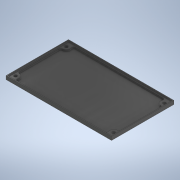
# Autodesk Inventor part: SUSTAINA-Core-Board_cover
Saved by Autodesk Inventor 2022.3 (Build 263350000, 350)
## iProperties
Part Number: SUSTAINA-Core-Board_cover
Material: 一般
Document SubType Name: Modeling
Designer: Masato Kubotera
Density: 1 g/cm^3
Appearance: 濃い灰色
Description: PLA
Mass: 6.13737 g
Surface Area: 193.634 cm^2
Volume: 6.13737 cm^3
Author: Masato Kubotera
Autodesk Inventor part; units mm, degrees
ref_plane "YZ Plane" through (0, 0, 0) normal (1, 0, 0) x (0, 1, 0)
ref_plane "XZ Plane" through (0, 0, 0) normal (0, 1, 0) x (-1, 0, 0)
derived "MainBoard.ipt"
sketch "スケッチ3" plane through (0, 0, -88.5) normal (0, 0, 1) x (1, 0, 0)
  line L0 (20.25, -135) -> (20.25, 0)
  line L1 (-83.25, 0) -> (-83.25, -135)
  line L2 (-31.5, -135) -> (-31.5, 0) construction
  line L3 (-83.25, -67.5) -> (20.25, -67.5) construction
  line L4 (-52.45, 1.4849) -> (-52.45, 5)
  line L5 (-52.45, 5) -> (-10.55, 5)
  line L6 (-10.55, 5) -> (-10.55, 1.4849)
  arc A0 (-53.9349, 0) -> (-52.45, 1.4849) centre (-53.1925, 0.7425) ccw
  arc A1 (-10.55, 1.4849) -> (-9.0651, 0) centre (-9.8075, 0.7425) ccw
  line L7 (-53.9349, 0) -> (-83.25, 0)
  line L8 (20.25, 0) -> (-9.0651, 0)
  line L9 (-10.55, 0) -> (-52.45, 0)
  line L10 (-52.45, -136.4849) -> (-52.45, -140)
  line L11 (-52.45, -140) -> (-10.55, -140)
  line L12 (-10.55, -140) -> (-10.55, -136.4849)
  arc A2 (-52.45, -136.4849) -> (-53.9349, -135) centre (-53.1925, -135.7425) ccw
  arc A3 (-9.0651, -135) -> (-10.55, -136.4849) centre (-9.8075, -135.7425) ccw
  line L13 (-53.9349, -135) -> (-83.25, -135)
  line L14 (20.25, -135) -> (-9.0651, -135)
  line L15 (-10.55, -135) -> (-52.45, -135)
  line L16 (18, -127.5) -> (-52, -127.5) construction
  line L17 (-52, -127.5) -> (-52, -7.5) construction
  line L18 (-52, -7.5) -> (18, -7.5) construction
  line L19 (18, -7.5) -> (18, -127.5) construction
  line L20 (18, -127.5) -> (-52, -7.5) construction
  line L21 (-52, -127.5) -> (18, -7.5) construction
  line L22 (-48.5, -116.5) -> (-48.5, -18.5)
  line L23 (-38.5627, -9.5) -> (4.5627, -9.5)
  line L24 (12.5, -10.5) -> (-46.5, -10.5) construction
  line L25 (-46.5, -10.5) -> (-46.5, -124.5) construction
  line L26 (-46.5, -124.5) -> (12.5, -124.5) construction
  line L27 (12.5, -124.5) -> (12.5, -10.5) construction
  line L28 (12.5, -10.5) -> (-46.5, -124.5) construction
  line L29 (-46.5, -10.5) -> (12.5, -124.5) construction
  circle A4 centre (12.5, -10.5) radius 2
  circle A5 centre (-46.5, -10.5) radius 2
  arc A6 (-46.5, -16.5) -> (-40.5471, -11.25) centre (-46.5, -10.5) ccw
  arc A7 (6.5471, -11.25) -> (12.5, -16.5) centre (12.5, -10.5) ccw
  line L30 (14.5, -18.5) -> (14.5, -116.5)
  line L31 (-17, -7.5) -> (-17, -127.5) construction
  line L32 (-76.25, -65) -> (-56.5, -65)
  line L33 (-54.5, -63) -> (-54.5, -7)
  line L34 (-56.5, -5) -> (-76.25, -5)
  line L35 (-78.25, -7) -> (-78.25, -63)
  arc A8 (-78.25, -63) -> (-76.25, -65) centre (-76.25, -63) ccw
  arc A9 (-56.5, -65) -> (-54.5, -63) centre (-56.5, -63) ccw
  arc A10 (-54.5, -7) -> (-56.5, -5) centre (-56.5, -7) ccw
  arc A11 (-76.25, -5) -> (-78.25, -7) centre (-76.25, -7) ccw
  arc A12 (-46.5, -16.5) -> (-48.5, -18.5) centre (-46.5, -18.5) ccw
  arc A13 (-38.5627, -9.5) -> (-40.5471, -11.25) centre (-38.5627, -11.5) ccw
  arc A14 (6.5471, -11.25) -> (4.5627, -9.5) centre (4.5627, -11.5) ccw
  arc A15 (14.5, -18.5) -> (12.5, -16.5) centre (12.5, -18.5) ccw
  line L36 (-38.5627, -125.5) -> (4.5627, -125.5)
  circle A16 centre (12.5, -124.5) radius 2
  circle A17 centre (-46.5, -124.5) radius 2
  arc A18 (-40.5471, -123.75) -> (-46.5, -118.5) centre (-46.5, -124.5) ccw
  arc A19 (12.5, -118.5) -> (6.5471, -123.75) centre (12.5, -124.5) ccw
  line L37 (-76.25, -70) -> (-56.5, -70)
  line L38 (-54.5, -72) -> (-54.5, -128)
  line L39 (-56.5, -130) -> (-76.25, -130)
  line L40 (-78.25, -128) -> (-78.25, -72)
  arc A20 (-76.25, -70) -> (-78.25, -72) centre (-76.25, -72) ccw
  arc A21 (-54.5, -72) -> (-56.5, -70) centre (-56.5, -72) ccw
  arc A22 (-56.5, -130) -> (-54.5, -128) centre (-56.5, -128) ccw
  arc A23 (-78.25, -128) -> (-76.25, -130) centre (-76.25, -128) ccw
  arc A24 (-48.5, -116.5) -> (-46.5, -118.5) centre (-46.5, -116.5) ccw
  arc A25 (-40.5471, -123.75) -> (-38.5627, -125.5) centre (-38.5627, -123.5) ccw
  arc A26 (4.5627, -125.5) -> (6.5471, -123.75) centre (4.5627, -123.5) ccw
  arc A27 (12.5, -118.5) -> (14.5, -116.5) centre (12.5, -116.5) ccw
  line L41 (12.5, -8.0316) -> (12.5, 3.8973)
  point P0 (0, 0)
  point P1 (-31.5, -67.5)
  point P2 (-17, -67.5)
  point P3 (-48.5, -16.1569)
  point P4 (-40.5839, -9.5)
  point P5 (6.5839, -9.5)
  point P6 (14.5, -16.1569)
sketch "スケッチ2" plane through (20.25, 0, -88.5) normal (0, 0, -1) x (0, -1, 0)
  line L0 (127.5, 72.25) -> (7.5, 72.25)
  line L1 (127.5, 2.25) -> (127.5, 72.25)
  line L2 (7.5, 72.25) -> (7.5, 2.25)
  line L3 (7.5, 2.25) -> (127.5, 2.25)
  circle A0 centre (10.5, 66.75) radius 2
  circle A1 centre (10.5, 7.75) radius 2
  circle A2 centre (124.5, 66.75) radius 2
  circle A3 centre (124.5, 7.75) radius 2
  circle A4 centre (10.5, 7.75) radius 1.6
  circle A5 centre (10.5, 66.75) radius 1.6
  circle A6 centre (124.5, 66.75) radius 1.6
  circle A7 centre (124.5, 7.75) radius 1.6
  arc A8 (120.3462, 68.4808) -> (124.5, 62.25) centre (124.5, 66.75) ccw
  line L4 (118.5, 71.25) -> (16.5, 71.25)
  line L5 (126.5, 60.25) -> (126.5, 14.25)
  line L6 (67.5, 103.5) -> (67.5, 0) construction
  line L7 (7.5, 37.25) -> (127.5, 37.25) construction
  arc A9 (10.5, 62.25) -> (14.6538, 68.4808) centre (10.5, 66.75) ccw
  arc A10 (124.5, 12.25) -> (120.3462, 6.0192) centre (124.5, 7.75) ccw
  arc A11 (14.6538, 6.0192) -> (10.5, 12.25) centre (10.5, 7.75) ccw
  line L8 (118.5, 3.25) -> (16.5, 3.25)
  line L9 (8.5, 14.25) -> (8.5, 60.25)
  arc A12 (120.3462, 68.4808) -> (118.5, 71.25) centre (118.5, 69.25) ccw
  arc A13 (126.5, 60.25) -> (124.5, 62.25) centre (124.5, 60.25) ccw
  arc A14 (124.5, 12.25) -> (126.5, 14.25) centre (124.5, 14.25) ccw
  arc A15 (118.5, 3.25) -> (120.3462, 6.0192) centre (118.5, 5.25) ccw
  arc A16 (14.6538, 6.0192) -> (16.5, 3.25) centre (16.5, 5.25) ccw
  arc A17 (8.5, 14.25) -> (10.5, 12.25) centre (10.5, 14.25) ccw
  arc A18 (10.5, 62.25) -> (8.5, 60.25) centre (10.5, 60.25) ccw
  arc A19 (16.5, 71.25) -> (14.6538, 68.4808) centre (16.5, 69.25) ccw
  point P0 (0, 20.25)
  point P1 (124.5, 71.25)
  point P2 (126.5, 62.7189)
  point P3 (10.5, 71.25)
  point P4 (126.5, 11.7811)
  point P5 (8.5, 62.7189)
  point P6 (124.5, 3.25)
  point P7 (8.5, 11.7811)
  point P8 (10.5, 3.25)
ref_plane "作業平面1" through (20.25, 0, -88.5) normal (0, 0, -1) x (0, -1, 0)
sketch "スケッチ4" plane through (20.25, 0, -88.5) normal (0, 0, -1) x (0, -1, 0)
  line L0 (6.25, 73.5) -> (128.75, 73.5)
  line L1 (128.75, 73.5) -> (128.75, 1)
  line L2 (128.75, 1) -> (6.25, 1)
  line L3 (6.25, 1) -> (6.25, 73.5)
  line L4 (6.25, 73.5) -> (128.75, 1) construction
  line L5 (128.75, 73.5) -> (6.25, 1) construction
  line L6 (7.25, 72.5) -> (127.75, 72.5)
  line L7 (127.75, 72.5) -> (127.75, 2)
  line L8 (127.75, 2) -> (7.25, 2)
  line L9 (7.25, 2) -> (7.25, 72.5)
  line L10 (7.25, 72.5) -> (127.75, 2) construction
  line L11 (127.75, 72.5) -> (7.25, 2) construction
  line L12 (7.5, 2.25) -> (127.5, 2.25) construction
  line L13 (7.5, 72.25) -> (7.5, 2.25) construction
  circle A0 centre (10.5, 7.75) radius 1.75
  circle A1 centre (10.5, 66.75) radius 1.75
  circle A2 centre (124.5, 7.75) radius 1.75
  circle A3 centre (124.5, 66.75) radius 1.75
  line L14 (118.5, 3.25) -> (16.5, 3.25) projected
  arc A4 (14.6538, 6.0192) -> (16.5, 3.25) centre (16.5, 5.25) ccw projected
  arc A5 (14.6538, 6.0192) -> (10.5, 12.25) centre (10.5, 7.75) ccw projected
  arc A6 (8.5, 14.25) -> (10.5, 12.25) centre (10.5, 14.25) ccw projected
  line L15 (8.5, 14.25) -> (8.5, 60.25) projected
  arc A7 (10.5, 62.25) -> (8.5, 60.25) centre (10.5, 60.25) ccw projected
  arc A8 (10.5, 62.25) -> (14.6538, 68.4808) centre (10.5, 66.75) ccw projected
  arc A9 (16.5, 71.25) -> (14.6538, 68.4808) centre (16.5, 69.25) ccw projected
  line L16 (118.5, 71.25) -> (16.5, 71.25) projected
  arc A10 (118.5, 3.25) -> (120.3462, 6.0192) centre (118.5, 5.25) ccw projected
  arc A11 (124.5, 12.25) -> (120.3462, 6.0192) centre (124.5, 7.75) ccw projected
  arc A12 (124.5, 12.25) -> (126.5, 14.25) centre (124.5, 14.25) ccw projected
  line L17 (126.5, 60.25) -> (126.5, 14.25) projected
  arc A13 (126.5, 60.25) -> (124.5, 62.25) centre (124.5, 60.25) ccw projected
  arc A14 (120.3462, 68.4808) -> (124.5, 62.25) centre (124.5, 66.75) ccw projected
  arc A15 (120.3462, 68.4808) -> (118.5, 71.25) centre (118.5, 69.25) ccw projected
  point P0 (0, 20.25)
  point P1 (67.5, 37.25)
  point P2 (67.5, 37.25)
  point P3 (67.5, 37.25)
  point P4 (67.5, 37.25)
  point P5 (10.5, 7.75)
  point P6 (124.5, 66.75)
  point P7 (124.5, 7.75)
  dimension "d5" = 1
  dimension "d6" = 1
  dimension "d7" = 0.25
  dimension "d8" = 0.25
  dimension "d11" = 3.5
  dimension "d12" = 3.5
  dimension "d13" = 3.5
  dimension "d14" = 3.5
  constraints: 24 end point, 6 midpoint, 5 coincident, 4 centre point, 4 parallel, 2 horizontal, 2 perpendicular
  measures "d5" distance between parallel lines of L2 L8
  measures "d6" distance between parallel lines of L3 L9
  measures "d7" distance between parallel lines of L8 L12
  measures "d8" distance between parallel lines of L13 L9
  measures "d11" diameter of A0
  measures "d12" diameter of A1
  measures "d13" diameter of A2
  measures "d14" diameter of A3
extrude "押し出し1" add sketch "スケッチ4" against normal blind 4 contours L0 L1 L2 L3
extrude "押し出し2" add sketch "スケッチ4" against normal blind 2.4 contours L6 L7 L8 L9
extrude "押し出し3" add sketch "スケッチ2" against normal blind 0.4 contours A8 A13 L5 A14 A10 A15 L8 A16 A11 A17 L9 A18 A9 A19 L4 A12
equation "\"d6\" = d5"
equation "\"d8\" = d7"
equation "\"d12\" = d11"
equation "\"d13\" = d11"
equation "\"d14\" = d11"
